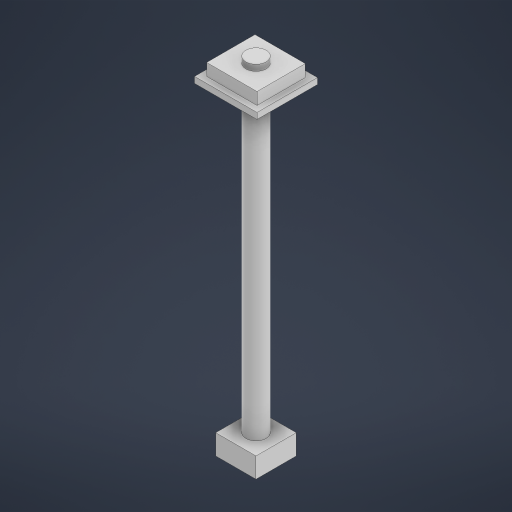
# Autodesk Inventor part: camera assembly
Saved by Autodesk Inventor 2024 (Build 280153000, 153)
## iProperties
Created: 2023-06-15
Part Number: camera assembly
Material: 일반
Document SubType Name: Modeling
Designer: 6gioc
Density: 1 g/cm^3
Appearance: 기본값
Author: 6gioc
Autodesk Inventor part; units mm, degrees
ref_plane "YZ Plane" through (0, 0, 0) normal (1, 0, 0) x (0, 1, 0)
ref_plane "XZ Plane" through (0, 0, 0) normal (0, 1, 0) x (-1, 0, 0)
ref_plane "XY Plane" through (0, 0, 0) normal (0, 0, 1) x (1, 0, 0)
sketch "스케치1" plane through (0, 0, 0) normal (0, 1, 0) x (-1, 0, 0)
  line L0 (0, 0) -> (25, 0)
  line L1 (25, 0) -> (25, -24)
  line L2 (25, -24) -> (0, -24)
  line L3 (0, -24) -> (0, 0)
  dimension "d0" = 25
  dimension "d1" = 24
  constraints: 8 end point, 2 parallel, 1 horizontal, 1 perpendicular
  measures "d0" distance of L1.end L2.end
  measures "d1" distance of L0.end L1.end
extrude "돌출1" add sketch "스케치1" along normal blind 9
sketch "스케치2" plane through (0, 9, 0) normal (0, 1, 0) x (1, 0, 0)
  line L0 (-25, 0) -> (0, 24) construction
  line L1 (-25, 24) -> (0, 0) construction
  circle A0 centre (-12.5, 12) radius 5.024
  circle A1 centre (-12.5, 12) radius 5.024
  line L2 (-25, 0) -> (0, 0)
  line L3 (0, 0) -> (0, 24)
  line L4 (0, 24) -> (-25, 24)
  line L5 (-25, 24) -> (-25, 0)
  constraints: 12 end point, 2 centre point, 2 parallel, 1 coincident, 1 concentric, 1 horizontal, 1 midpoint, 1 perpendicular
extrude "돌출2" cut sketch "스케치2" against normal blind 3
sketch "스케치3" plane through (0, 0, 0) normal (0, -1, 0) x (1, 0, 0)
  line L0 (-28, -27) -> (3, -27)
  line L1 (3, -27) -> (3, 3)
  line L2 (3, 3) -> (-28, 3)
  line L3 (-28, 3) -> (-28, -27)
  line L4 (-25, -24) -> (-25, 0) projected
  line L5 (-25, 0) -> (0, 0) projected
  line L6 (0, -24) -> (-25, -24) projected
  line L7 (0, 0) -> (0, -24) projected
  dimension "d6" = 3
  dimension "d7" = 3
  dimension "d8" = 3
  dimension "d9" = 3
  constraints: 8 end point, 2 parallel, 1 horizontal, 1 perpendicular
  measures "d6" distance between parallel lines of L3 L4
  measures "d7" distance between parallel lines of L5 L2
  measures "d8" distance between parallel lines of L0 L6
  measures "d9" distance between parallel lines of L1 L7
extrude "돌출3" add sketch "스케치3" along normal blind 3 separate body contours L3 L2 L1 L0 | L4 L5 L7 L6
sketch "스케치4" plane through (0, -3, 0) normal (0, -1, 0) x (1, 0, 0)
  line L0 (-28, 3) -> (-28, -27) projected
  line L1 (-28, -27) -> (3.0102, 3)
  line L2 (3, -27) -> (3, 3) projected
  line L3 (3, -27) -> (-28, 3)
  circle A0 centre (-12.5, -12) radius 5
  point P0 (0, 0)
  dimension "d12" = 10
  constraints: 4 end point, 1 centre point, 1 midpoint
  measures "d12" diameter of A0
extrude "돌출4" add sketch "스케치4" along normal blind 150 separate body contours A0 L1 L3 | L3 L1 A0 | L1 L3 A0 | L1 A0 L3
sketch "스케치5" plane through (-12.5, -153, -12) normal (0, -1, 0) x (1, 0, 0)
  line L0 (0, 0) -> (10, 0)
  line L1 (10, 0) -> (10, -10)
  line L2 (10, -10) -> (0, -10)
  line L3 (0, -10) -> (0, 0)
  line L4 (10, -10) -> (-10, -10)
  line L5 (-10, -10) -> (-10, 10)
  line L6 (-10, 10) -> (10, 10)
  line L7 (10, 10) -> (10, -10)
  point P0 (12.5, 12)
  dimension "d15" = 10
  dimension "d16" = 10
  dimension "d17" = 20
  dimension "d18" = 20
  constraints: 16 end point, 4 parallel, 2 horizontal, 2 perpendicular
  measures "d15" distance of L1.end L2.end
  measures "d16" distance of L0.end L1.end
  measures "d17" distance of L5.end L6.end
  measures "d18" distance of L4.end L5.end
extrude "돌출5" add sketch "스케치5" along normal blind 10 separate body
sketch "스케치6" plane through (-22.5, -153, -22) normal (-1, 0, 0) x (0, 0, 1)
  line L0 (0, -10) -> (20, -10) projected
  line L1 (0, 0) -> (20, -10)
  line L2 (0, 0) -> (20, 0) projected
  line L3 (20, 0) -> (0, -10)
  circle A0 centre (10, -5) radius 2.5
  circle A1 centre (10, -5) radius 1.5
  line L4 (10, -5) -> (8.5905, -4.487)
  line L5 (10, -5) -> (11.5, -5) construction
  line L6 (8.5905, -4.487) -> (7.9064, -6.3664)
  line L7 (8.5905, -4.487) -> (9.2745, -2.6076)
  line L8 (10, -5) -> (11.4095, -5.513)
  line L9 (11.4095, -5.513) -> (12.0936, -3.6336)
  line L10 (11.4095, -5.513) -> (10.7255, -7.3924)
  point P0 (22, 153)
  point P1 (8.6584, -4.3292)
  point P2 (11.3505, -5.6752)
  point P3 (11.3416, -5.6708)
  point P4 (8.6495, -4.3248)
  dimension "d21" = 5
  dimension "d22" = 3
  dimension "d23" = 160
  constraints: 18 end point, 6 point on circle, 2 centre point, 2 perpendicular, 1 coincident, 1 equal length, 1 horizontal, 1 midpoint, 1 point on line
  measures "d21" diameter of A0
  measures "d22" diameter of A1
  measures "d23" angle of L5 L4
extrude "돌출6" cut sketch "스케치6" against normal blind 5 contours L6 A1 L3 | L3 A1 L1 L10 A0 L6 | A1 L4 L3 | L3 L1 A1 | A1 L1 L4 | L7 A0 L9 L3 A1 L1 | L1 L8 A1 | L8 L3 A1 | A1 L3 L9 | L1 A1 L3 bodies 4
